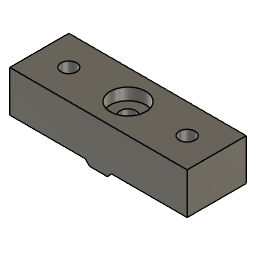
Gantry to Frame Bracket (Autodesk Fusion 360 design; units mm, degrees)
part number: 2026-06-20-21-18-59-522
Autodesk Fusion 360 part; units mm, degrees
sketch "Sketch1" plane through (0, 0, 0) normal (0, 0, 1) x (1, 0, 0)
  line L0 (30, -10) -> (-30, -10)
  line L1 (-30, -10) -> (-30, 10)
  line L2 (-30, 10) -> (30, 10)
  line L3 (30, 10) -> (30, -10)
  line L4 (30, -10) -> (-30, 10) construction
  line L5 (-30, -10) -> (30, 10) construction
  circle A0 centre (0, 0) radius 2.65
  circle A1 centre (20, 0) radius 2.65
  circle A2 centre (-20, 0) radius 2.65
  circle A3 centre (-20, 0) radius 6
  circle A4 centre (20, 0) radius 6
  dimension "d1" = 60
  dimension "d2" = 20
  dimension "d3" = 5.3
  dimension "d4" = 5.3
  dimension "d5" = 5.3
  dimension "d11" = 12
  dimension "d12" = 12
  constraint horizontal L0
  constraint perpendicular L0 L1
  constraint parallel L0 L2
  constraint parallel L1 L3
  constraint coincident L4 A0.centre
  constraint coincident L5 A0.centre
  constraint coincident A0.centre origin
  constraint concentric A2 A3
  constraint concentric A1 A4
  measures "d1" distance of L1.end L2.end
  measures "d2" distance of L0.end L1.end
  measures "d3" diameter of A0
  measures "d4" diameter of A1
  measures "d5" diameter of A2
  measures "d11" diameter of A3
  measures "d12" diameter of A4
extrude "Extrude1" add sketch "Sketch1" along normal blind 6 contours L0 L1 L2 L3 | A3 | A4
sketch "Sketch2" plane through (0, 0, 6) normal (0, 0, 1) x (-1, 0, 0)
  circle A0 centre (0, 0) radius 2.65
  circle A1 centre (-20, 0) radius 2.65
  circle A2 centre (20, 0) radius 2.65
  line L0 (-30, -10) -> (30, -10)
  line L1 (30, -10) -> (30, 10)
  line L2 (30, 10) -> (-30, 10)
  line L3 (-30, 10) -> (-30, -10)
  circle A3 centre (0, 0) radius 6
  dimension "d8" = 12
  constraint coincident A0.centre A3.centre
  measures "d8" diameter of A3
extrude "Extrude2" add sketch "Sketch2" along normal blind 4 contours L0 L1 L2 L3
extrude "Extrude4" add sketch "Sketch1" against normal blind 4 contours L0 L1 L2 L3
sketch "Sketch3" plane through (0, 0, -4) normal (0, 0, -1) x (1, 0, 0)
  circle A0 centre (0, 0) radius 2.65
  circle A1 centre (20, 0) radius 6
  circle A2 centre (-20, 0) radius 6
  line L0 (-30, -10) -> (30, -10)
  line L1 (30, -10) -> (30, 10)
  line L2 (30, 10) -> (-30, 10)
  line L3 (-30, 10) -> (-30, -10)
  line L4 (-4.5, 5) -> (4.5, 5)
  line L5 (4.5, 5) -> (4.5, 10)
  line L6 (4.5, 10) -> (-4.5, 10)
  line L7 (-4.5, 10) -> (-4.5, 5)
  line L8 (-4.5, -10) -> (4.5, -10)
  line L9 (4.5, -10) -> (4.5, -5)
  line L10 (4.5, -5) -> (-4.5, -5)
  line L11 (-4.5, -5) -> (-4.5, -10)
  dimension "d17" = 9
  dimension "d18" = 5
  dimension "d19" = 9
  dimension "d20" = 5
  constraint horizontal L4
  constraint vertical L5
  constraint horizontal L6
  constraint vertical L7
  constraint midpoint L2 L6
  constraint horizontal L8
  constraint vertical L9
  constraint horizontal L10
  constraint vertical L11
  constraint midpoint L0 L8
  measures "d17" distance of L4.start L4.end
  measures "d18" distance of L4.start L6.end
  measures "d19" distance of L8.start L8.end
  measures "d20" distance of L8.start L10.end
extrude "Extrude5" add sketch "Sketch3" along normal blind 1.5 contours L0 L8 L9 L10 L11 | L2 L4 L5 L6 L7
chamfer "Chamfer1" distance 1.5 angle 45 6 edges at (-4.5, -7.5, -5.5) (0, -5, -5.5) (4.5, -7.5, -5.5) (-4.5, 7.5, -5.5) (0, 5, -5.5) (4.5, 7.5, -5.5)
extrude "Extrude3" [suppressed]
named bodies: "Ganrty to Frame Bracket"
